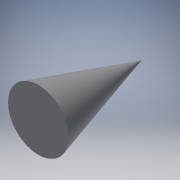
# Autodesk Inventor part: cone
Saved by Autodesk Inventor 2018 (Build 220112000, 112)
## iProperties
Created: 2018-04-02
Part Number: cone
Material: ABS plástico
Document SubType Name: Modeling
Designer: Ernandes
Density: 1.06 g/cm^3
Appearance: Liso - Branco
Mass: 6.55361 g
Surface Area: 20.629 cm^2
Volume: 6.18265 cm^3
Author: Ernandes
Autodesk Inventor part; units mm, degrees
ref_plane "YZ Plane" through (0, 0, 0) normal (1, 0, 0) x (0, 1, 0)
ref_plane "XZ Plane" through (0, 0, 0) normal (0, 1, 0) x (-1, 0, 0)
ref_plane "XY Plane" through (0, 0, 0) normal (0, 0, 1) x (1, 0, 0)
sketch "Esboço1" plane through (0, 0, 0) normal (0, 0, 1) x (1, 0, 0)
  line L0 (0, 0) -> (12, 0)
  line L1 (0, 0) -> (0, 41)
  line L2 (0, 41) -> (12, 0)
  dimension "d0" = 12
  dimension "d1" = 41
  constraints: 6 end point, 1 horizontal, 1 vertical
  measures "d0" distance of L0.start L0.end
  measures "d1" distance of L0.start L1.end
revolve "Revolução1" add sketch "Esboço1" angle 360 about axis through (0, 0, 0) along (0, 1, 0)
